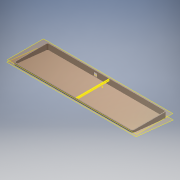
# Autodesk Inventor part: FullEnclosurePrototype
Saved by Autodesk Inventor 2016 (Build 200138000, 138)
## iProperties
Created: 2021-04-05
Part Number: FullEnclosurePrototype
Material: Generic
Document SubType Name: Modeling
Designer: Tom
Density: 1 g/cm^3
Appearance: Default
Author: Tom
Autodesk Inventor part; units mm, degrees
ref_plane "YZ Plane" through (0, 0, 0) normal (1, 0, 0) x (0, 1, 0)
ref_plane "XZ Plane" through (0, 0, 0) normal (0, 1, 0) x (-1, 0, 0)
ref_plane "XY Plane" through (0, 0, 0) normal (0, 0, 1) x (1, 0, 0)
sketch "Sketch1" plane through (0, 0, 0) normal (1, 0, 0) x (0, 1, 0)
  line L0 (-93.1541, 14.0981) -> (20.8459, 14.0981) projected
  line L1 (-93.1541, 14.0981) -> (-93.1541, 12.5981) projected
  line L2 (20.8459, 12.5981) -> (-93.1541, 12.5981) projected
  line L3 (20.8459, 14.0981) -> (20.8459, 12.5981) projected
  line L4 (-93.1541, 7.4943) -> (-93.1541, 9.0943) projected
  line L5 (-93.1541, 7.4943) -> (20.8459, 7.4943) projected
  line L6 (20.8459, 7.4943) -> (20.8459, 9.0943) projected
  line L7 (-93.1541, 9.0943) -> (20.8459, 9.0943) projected
  line L8 (25.5959, 14.0981) -> (20.8459, 14.0981) projected
  line L9 (20.8459, 12.5981) -> (25.5959, 12.5981) projected
  line L10 (25.5959, 14.0981) -> (25.5959, 12.5981) projected
  line L11 (25.5959, 9.0943) -> (20.8459, 9.0943) projected
  line L12 (25.5959, 7.4943) -> (20.8459, 7.4943) projected
  line L13 (25.5959, 7.4943) -> (25.5959, 9.0943) projected
  line L14 (-93.1541, 9.0943) -> (-97.9041, 9.0943) projected
  line L15 (-93.1541, 7.4943) -> (-97.9041, 7.4943) projected
  line L16 (-97.9041, 7.4943) -> (-97.9041, 9.0943) projected
  line L17 (-93.1541, 14.0981) -> (-97.9041, 14.0981) projected
  line L18 (-97.9041, 12.5981) -> (-93.1541, 12.5981) projected
  line L19 (-97.9041, 14.0981) -> (-97.9041, 12.5981) projected
  line L20 (-93.4041, 11.6343) -> (-93.3041, 11.6343) projected
  point P0 (0, 0)
ref_plane "Work Plane1" through (-45.4451, 14.3376, -5.5632) normal (0, 0.1062088, 0.9943439) x (-1, 0, 0)
ref_plane "Work Plane2" through (-9.3413, -36.1541, 14.0981) normal (0, 0, 1) x (1, 0, 0)
sketch "Sketch3" plane through (-9.3413, -36.1541, 14.0981) normal (0, 0, 1) x (1, 0, 0)
  line L0 (-211.6644, 41.535) -> (-205.2313, 59.21) projected
  line L1 (-205.2313, 59.21) -> (-202.7313, 59.21) projected
  line L2 (-202.7313, 59.21) -> (-209.1644, 41.535) projected
  line L3 (-209.1644, 41.535) -> (-211.6644, 41.535) projected
  line L4 (-201.6644, 41.535) -> (-195.2313, 59.21) projected
  line L5 (-195.2313, 59.21) -> (-192.7313, 59.21) projected
  line L6 (-192.7313, 59.21) -> (-199.1644, 41.535) projected
  line L7 (-199.1644, 41.535) -> (-201.6644, 41.535) projected
  line L8 (-191.6644, 41.535) -> (-185.2313, 59.21) projected
  line L9 (-185.2313, 59.21) -> (-182.7313, 59.21) projected
  line L10 (-182.7313, 59.21) -> (-189.1644, 41.535) projected
  line L11 (-189.1644, 41.535) -> (-191.6644, 41.535) projected
  line L12 (-181.6644, 41.535) -> (-175.2313, 59.21) projected
  line L13 (-175.2313, 59.21) -> (-172.7313, 59.21) projected
  line L14 (-172.7313, 59.21) -> (-179.1644, 41.535) projected
  line L15 (-179.1644, 41.535) -> (-181.6644, 41.535) projected
  line L16 (-171.6644, 41.535) -> (-165.2313, 59.21) projected
  line L17 (-165.2313, 59.21) -> (-162.7313, 59.21) projected
  line L18 (-162.7313, 59.21) -> (-169.1644, 41.535) projected
  line L19 (-169.1644, 41.535) -> (-171.6644, 41.535) projected
  line L20 (-161.6644, 41.535) -> (-155.2313, 59.21) projected
  line L21 (-155.2313, 59.21) -> (-152.7313, 59.21) projected
  line L22 (-152.7313, 59.21) -> (-159.1644, 41.535) projected
  line L23 (-159.1644, 41.535) -> (-161.6644, 41.535) projected
  line L24 (-151.6644, 41.535) -> (-145.2313, 59.21) projected
  line L25 (-145.2313, 59.21) -> (-142.7313, 59.21) projected
  line L26 (-142.7313, 59.21) -> (-149.1644, 41.535) projected
  line L27 (-149.1644, 41.535) -> (-151.6644, 41.535) projected
  line L28 (-141.6644, 41.535) -> (-135.2313, 59.21) projected
  line L29 (-135.2313, 59.21) -> (-132.7313, 59.21) projected
  line L30 (-132.7313, 59.21) -> (-139.1644, 41.535) projected
  line L31 (-139.1644, 41.535) -> (-141.6644, 41.535) projected
  line L32 (-134.1647, 41.535) -> (-136.6647, 41.535) projected
  line L33 (-136.6647, 41.535) -> (-131.39, 56.027) projected
  line L34 (-131.39, 56.027) -> (-131.39, 49.1583) projected
  line L35 (-131.39, 49.1583) -> (-134.1647, 41.535) projected
  line L36 (-141.27, 35.75) -> (-143.77, 35.75) projected
  line L37 (-143.77, 35.75) -> (-142.3378, 39.685) projected
  line L38 (-142.3378, 39.685) -> (-139.8378, 39.685) projected
  line L39 (-139.8378, 39.685) -> (-141.27, 35.75) projected
  line L40 (-151.27, 35.75) -> (-153.77, 35.75) projected
  line L41 (-153.77, 35.75) -> (-152.3378, 39.685) projected
  line L42 (-152.3378, 39.685) -> (-149.8378, 39.685) projected
  line L43 (-149.8378, 39.685) -> (-151.27, 35.75) projected
  line L44 (-161.27, 35.75) -> (-163.77, 35.75) projected
  line L45 (-163.77, 35.75) -> (-162.3378, 39.685) projected
  line L46 (-162.3378, 39.685) -> (-159.8378, 39.685) projected
  line L47 (-159.8378, 39.685) -> (-161.27, 35.75) projected
  line L48 (-171.27, 35.75) -> (-173.77, 35.75) projected
  line L49 (-173.77, 35.75) -> (-172.3378, 39.685) projected
  line L50 (-172.3378, 39.685) -> (-169.8378, 39.685) projected
  line L51 (-169.8378, 39.685) -> (-171.27, 35.75) projected
  line L52 (-181.27, 35.75) -> (-183.77, 35.75) projected
  line L53 (-183.77, 35.75) -> (-182.3378, 39.685) projected
  line L54 (-182.3378, 39.685) -> (-179.8378, 39.685) projected
  line L55 (-179.8378, 39.685) -> (-181.27, 35.75) projected
  line L56 (-191.27, 35.75) -> (-193.77, 35.75) projected
  line L57 (-193.77, 35.75) -> (-192.3378, 39.685) projected
  line L58 (-192.3378, 39.685) -> (-189.8378, 39.685) projected
  line L59 (-189.8378, 39.685) -> (-191.27, 35.75) projected
  line L60 (-201.27, 35.75) -> (-203.77, 35.75) projected
  line L61 (-203.77, 35.75) -> (-202.3378, 39.685) projected
  line L62 (-202.3378, 39.685) -> (-199.8378, 39.685) projected
  line L63 (-199.8378, 39.685) -> (-201.27, 35.75) projected
  line L64 (-211.27, 35.75) -> (-213.77, 35.75) projected
  line L65 (-213.77, 35.75) -> (-212.3378, 39.685) projected
  line L66 (-212.3378, 39.685) -> (-209.8378, 39.685) projected
  line L67 (-209.8378, 39.685) -> (-211.27, 35.75) projected
  line L68 (-206.27, 35.75) -> (-208.77, 35.75) projected
  line L69 (-208.77, 35.75) -> (-207.3378, 39.685) projected
  line L70 (-207.3378, 39.685) -> (-204.8378, 39.685) projected
  line L71 (-204.8378, 39.685) -> (-206.27, 35.75) projected
  line L72 (-196.27, 35.75) -> (-198.77, 35.75) projected
  line L73 (-198.77, 35.75) -> (-197.3378, 39.685) projected
  line L74 (-197.3378, 39.685) -> (-194.8378, 39.685) projected
  line L75 (-194.8378, 39.685) -> (-196.27, 35.75) projected
  line L76 (-186.27, 35.75) -> (-188.77, 35.75) projected
  line L77 (-188.77, 35.75) -> (-187.3378, 39.685) projected
  line L78 (-187.3378, 39.685) -> (-184.8378, 39.685) projected
  line L79 (-184.8378, 39.685) -> (-186.27, 35.75) projected
  line L80 (-176.27, 35.75) -> (-178.77, 35.75) projected
  line L81 (-178.77, 35.75) -> (-177.3378, 39.685) projected
  line L82 (-177.3378, 39.685) -> (-174.8378, 39.685) projected
  line L83 (-174.8378, 39.685) -> (-176.27, 35.75) projected
  line L84 (-166.27, 35.75) -> (-168.77, 35.75) projected
  line L85 (-168.77, 35.75) -> (-167.3378, 39.685) projected
  line L86 (-167.3378, 39.685) -> (-164.8378, 39.685) projected
  line L87 (-164.8378, 39.685) -> (-166.27, 35.75) projected
  line L88 (-156.27, 35.75) -> (-158.77, 35.75) projected
  line L89 (-158.77, 35.75) -> (-157.3378, 39.685) projected
  line L90 (-157.3378, 39.685) -> (-154.8378, 39.685) projected
  line L91 (-154.8378, 39.685) -> (-156.27, 35.75) projected
  line L92 (-146.27, 35.75) -> (-148.77, 35.75) projected
  line L93 (-148.77, 35.75) -> (-147.3378, 39.685) projected
  line L94 (-147.3378, 39.685) -> (-144.8378, 39.685) projected
  line L95 (-144.8378, 39.685) -> (-146.27, 35.75) projected
  line L96 (-136.2702, 35.75) -> (-138.7702, 35.75) projected
  line L97 (-138.7702, 35.75) -> (-137.338, 39.685) projected
  line L98 (-137.338, 39.685) -> (-134.838, 39.685) projected
  line L99 (-134.838, 39.685) -> (-136.2702, 35.75) projected
  line L100 (-213.77, 49.4867) -> (-210.231, 59.21) projected
  line L101 (-210.231, 59.21) -> (-207.731, 59.21) projected
  line L102 (-207.731, 59.21) -> (-213.77, 42.618) projected
  line L103 (-213.77, 42.618) -> (-213.77, 49.4867) projected
  line L104 (-146.6644, 41.535) -> (-140.2313, 59.21) projected
  line L105 (-140.2313, 59.21) -> (-137.7313, 59.21) projected
  line L106 (-137.7313, 59.21) -> (-144.1644, 41.535) projected
  line L107 (-144.1644, 41.535) -> (-146.6644, 41.535) projected
  line L108 (-156.6644, 41.535) -> (-150.2313, 59.21) projected
  line L109 (-150.2313, 59.21) -> (-147.7313, 59.21) projected
  line L110 (-147.7313, 59.21) -> (-154.1644, 41.535) projected
  line L111 (-154.1644, 41.535) -> (-156.6644, 41.535) projected
  line L112 (-166.6644, 41.535) -> (-160.2313, 59.21) projected
  line L113 (-160.2313, 59.21) -> (-157.7313, 59.21) projected
  line L114 (-157.7313, 59.21) -> (-164.1644, 41.535) projected
  line L115 (-164.1644, 41.535) -> (-166.6644, 41.535) projected
  line L116 (-176.6644, 41.535) -> (-170.2313, 59.21) projected
  line L117 (-170.2313, 59.21) -> (-167.7313, 59.21) projected
  line L118 (-167.7313, 59.21) -> (-174.1644, 41.535) projected
  line L119 (-174.1644, 41.535) -> (-176.6644, 41.535) projected
  line L120 (-186.6644, 41.535) -> (-180.2313, 59.21) projected
  line L121 (-180.2313, 59.21) -> (-177.7313, 59.21) projected
  line L122 (-177.7313, 59.21) -> (-184.1644, 41.535) projected
  line L123 (-184.1644, 41.535) -> (-186.6644, 41.535) projected
  line L124 (-196.6644, 41.535) -> (-190.2313, 59.21) projected
  line L125 (-190.2313, 59.21) -> (-187.7313, 59.21) projected
  line L126 (-187.7313, 59.21) -> (-194.1644, 41.535) projected
  line L127 (-194.1644, 41.535) -> (-196.6644, 41.535) projected
  line L128 (-206.6644, 41.535) -> (-200.2313, 59.21) projected
  line L129 (-200.2313, 59.21) -> (-197.7313, 59.21) projected
  line L130 (-197.7313, 59.21) -> (-204.1644, 41.535) projected
  line L131 (-204.1644, 41.535) -> (-206.6644, 41.535) projected
  line L132 (-78.7722, 35.75) -> (-133.77, 35.75) projected
  line L133 (-133.77, 35.75) -> (-132.3378, 39.685) projected
  line L134 (-132.3378, 39.685) -> (-77.34, 39.685) projected
  line L135 (-77.34, 39.685) -> (-78.7722, 35.75) projected
  line L136 (-77.34, 41.535) -> (-129.54, 41.535) projected
  line L137 (-129.54, 41.535) -> (-129.54, 59.315) projected
  line L138 (-129.54, 59.315) -> (-77.34, 59.315) projected
  line L139 (-77.34, 59.315) -> (-77.34, 41.535) projected
  line L140 (159, -26.25) -> (159, -40.25) projected
  line L141 (159, -40.25) -> (145, -40.25) projected
  line L142 (145, -40.25) -> (145, -26.25) projected
  line L143 (145, -26.25) -> (159, -26.25) projected
  line L144 (140, -26.25) -> (140, -40.25) projected
  line L145 (140, -40.25) -> (126, -40.25) projected
  line L146 (126, -40.25) -> (126, -26.25) projected
  line L147 (126, -26.25) -> (140, -26.25) projected
  line L148 (121, -26.25) -> (121, -40.25) projected
  line L149 (121, -40.25) -> (107, -40.25) projected
  line L150 (107, -40.25) -> (107, -26.25) projected
  line L151 (107, -26.25) -> (121, -26.25) projected
  line L152 (102, -26.25) -> (102, -40.25) projected
  line L153 (102, -40.25) -> (88, -40.25) projected
  line L154 (88, -40.25) -> (88, -26.25) projected
  line L155 (88, -26.25) -> (102, -26.25) projected
  line L156 (83, -26.25) -> (83, -40.25) projected
  line L157 (83, -40.25) -> (69, -40.25) projected
  line L158 (69, -40.25) -> (69, -26.25) projected
  line L159 (69, -26.25) -> (83, -26.25) projected
  line L160 (64, -26.25) -> (64, -40.25) projected
  line L161 (64, -40.25) -> (50, -40.25) projected
  line L162 (50, -40.25) -> (50, -26.25) projected
  line L163 (50, -26.25) -> (64, -26.25) projected
  line L164 (45, -26.25) -> (45, -40.25) projected
  line L165 (45, -40.25) -> (31, -40.25) projected
  line L166 (31, -40.25) -> (31, -26.25) projected
  line L167 (31, -26.25) -> (45, -26.25) projected
  line L168 (26, -26.25) -> (26, -40.25) projected
  line L169 (26, -40.25) -> (12, -40.25) projected
  line L170 (12, -40.25) -> (12, -26.25) projected
  line L171 (12, -26.25) -> (26, -26.25) projected
  line L172 (7, -26.25) -> (7, -40.25) projected
  line L173 (7, -40.25) -> (-7, -40.25) projected
  line L174 (-7, -40.25) -> (-7, -26.25) projected
  line L175 (-7, -26.25) -> (7, -26.25) projected
  line L176 (154.5, -7.25) -> (168.5, -7.25) projected
  line L177 (168.5, -7.25) -> (168.5, -21.25) projected
  line L178 (168.5, -21.25) -> (154.5, -21.25) projected
  line L179 (154.5, -21.25) -> (154.5, -7.25) projected
  line L180 (135.5, -7.25) -> (149.5, -7.25) projected
  line L181 (149.5, -7.25) -> (149.5, -21.25) projected
  line L182 (149.5, -21.25) -> (135.5, -21.25) projected
  line L183 (135.5, -21.25) -> (135.5, -7.25) projected
  line L184 (116.5, -7.25) -> (130.5, -7.25) projected
  line L185 (130.5, -7.25) -> (130.5, -21.25) projected
  line L186 (130.5, -21.25) -> (116.5, -21.25) projected
  line L187 (116.5, -21.25) -> (116.5, -7.25) projected
  line L188 (97.5, -7.25) -> (111.5, -7.25) projected
  line L189 (111.5, -7.25) -> (111.5, -21.25) projected
  line L190 (111.5, -21.25) -> (97.5, -21.25) projected
  line L191 (97.5, -21.25) -> (97.5, -7.25) projected
  line L192 (78.5, -7.25) -> (92.5, -7.25) projected
  line L193 (92.5, -7.25) -> (92.5, -21.25) projected
  line L194 (92.5, -21.25) -> (78.5, -21.25) projected
  line L195 (78.5, -21.25) -> (78.5, -7.25) projected
  line L196 (59.5, -7.25) -> (73.5, -7.25) projected
  line L197 (73.5, -7.25) -> (73.5, -21.25) projected
  line L198 (73.5, -21.25) -> (59.5, -21.25) projected
  line L199 (59.5, -21.25) -> (59.5, -7.25) projected
  line L200 (40.5, -7.25) -> (54.5, -7.25) projected
  line L201 (54.5, -7.25) -> (54.5, -21.25) projected
  line L202 (54.5, -21.25) -> (40.5, -21.25) projected
  line L203 (40.5, -21.25) -> (40.5, -7.25) projected
  line L204 (21.5, -7.25) -> (35.5, -7.25) projected
  line L205 (35.5, -7.25) -> (35.5, -21.25) projected
  line L206 (35.5, -21.25) -> (21.5, -21.25) projected
  line L207 (21.5, -21.25) -> (21.5, -7.25) projected
  line L208 (2.5, -7.25) -> (16.5, -7.25) projected
  line L209 (16.5, -7.25) -> (16.5, -21.25) projected
  line L210 (16.5, -21.25) -> (2.5, -21.25) projected
  line L211 (2.5, -21.25) -> (2.5, -7.25) projected
  line L212 (-16.5, -7.25) -> (-2.5, -7.25) projected
  line L213 (-2.5, -7.25) -> (-2.5, -21.25) projected
  line L214 (-2.5, -21.25) -> (-16.5, -21.25) projected
  line L215 (-16.5, -21.25) -> (-16.5, -7.25) projected
  line L216 (182.75, 11.75) -> (182.75, -2.25) projected
  line L217 (182.75, -2.25) -> (168.75, -2.25) projected
  line L218 (168.75, -2.25) -> (168.75, 11.75) projected
  line L219 (168.75, 11.75) -> (182.75, 11.75) projected
  line L220 (163.75, 11.75) -> (163.75, -2.25) projected
  line L221 (163.75, -2.25) -> (149.75, -2.25) projected
  line L222 (149.75, -2.25) -> (149.75, 11.75) projected
  line L223 (149.75, 11.75) -> (163.75, 11.75) projected
  line L224 (144.75, 11.75) -> (144.75, -2.25) projected
  line L225 (144.75, -2.25) -> (130.75, -2.25) projected
  line L226 (130.75, -2.25) -> (130.75, 11.75) projected
  line L227 (130.75, 11.75) -> (144.75, 11.75) projected
  line L228 (125.75, 11.75) -> (125.75, -2.25) projected
  line L229 (125.75, -2.25) -> (111.75, -2.25) projected
  line L230 (111.75, -2.25) -> (111.75, 11.75) projected
  line L231 (111.75, 11.75) -> (125.75, 11.75) projected
  line L232 (106.75, 11.75) -> (106.75, -2.25) projected
  line L233 (106.75, -2.25) -> (92.75, -2.25) projected
  line L234 (92.75, -2.25) -> (92.75, 11.75) projected
  line L235 (92.75, 11.75) -> (106.75, 11.75) projected
  line L236 (87.75, 11.75) -> (87.75, -2.25) projected
  line L237 (87.75, -2.25) -> (73.75, -2.25) projected
  line L238 (73.75, -2.25) -> (73.75, 11.75) projected
  line L239 (73.75, 11.75) -> (87.75, 11.75) projected
  line L240 (68.75, 11.75) -> (68.75, -2.25) projected
  line L241 (68.75, -2.25) -> (54.75, -2.25) projected
  line L242 (54.75, -2.25) -> (54.75, 11.75) projected
  line L243 (54.75, 11.75) -> (68.75, 11.75) projected
  line L244 (49.75, 11.75) -> (49.75, -2.25) projected
  line L245 (49.75, -2.25) -> (35.75, -2.25) projected
  line L246 (35.75, -2.25) -> (35.75, 11.75) projected
  line L247 (35.75, 11.75) -> (49.75, 11.75) projected
  line L248 (30.75, 11.75) -> (30.75, -2.25) projected
  line L249 (30.75, -2.25) -> (16.75, -2.25) projected
  line L250 (16.75, -2.25) -> (16.75, 11.75) projected
  line L251 (16.75, 11.75) -> (30.75, 11.75) projected
  line L252 (11.75, 11.75) -> (11.75, -2.25) projected
  line L253 (11.75, -2.25) -> (-2.25, -2.25) projected
  line L254 (-2.25, -2.25) -> (-2.25, 11.75) projected
  line L255 (-2.25, 11.75) -> (11.75, 11.75) projected
  line L256 (-7.25, 11.75) -> (-7.25, -2.25) projected
  line L257 (-7.25, -2.25) -> (-21.25, -2.25) projected
  line L258 (-21.25, -2.25) -> (-21.25, 11.75) projected
  line L259 (-21.25, 11.75) -> (-7.25, 11.75) projected
  line L260 (-12, -26.25) -> (-12, -40.25) projected
  line L261 (-12, -40.25) -> (-26, -40.25) projected
  line L262 (-26, -40.25) -> (-26, -26.25) projected
  line L263 (-26, -26.25) -> (-12, -26.25) projected
  line L264 (-21.5, -7.25) -> (-21.5, -21.25) projected
  line L265 (-21.5, -21.25) -> (-35.5, -21.25) projected
  line L266 (-35.5, -21.25) -> (-35.5, -7.25) projected
  line L267 (-35.5, -7.25) -> (-21.5, -7.25) projected
  line L268 (-26.25, 11.75) -> (-26.25, -2.25) projected
  line L269 (-26.25, -2.25) -> (-40.25, -2.25) projected
  line L270 (-40.25, -2.25) -> (-40.25, 11.75) projected
  line L271 (-40.25, 11.75) -> (-26.25, 11.75) projected
  line L272 (201.75, 30.75) -> (201.75, 16.75) projected
  line L273 (201.75, 16.75) -> (187.75, 16.75) projected
  line L274 (187.75, 16.75) -> (187.75, 30.75) projected
  line L275 (187.75, 30.75) -> (201.75, 30.75) projected
  line L276 (206.5, 11.75) -> (206.5, -2.25) projected
  line L277 (206.5, -2.25) -> (192.5, -2.25) projected
  line L278 (192.5, -2.25) -> (192.5, 11.75) projected
  line L279 (192.5, 11.75) -> (206.5, 11.75) projected
  line L280 (199.375, -7.25) -> (199.375, -21.25) projected
  line L281 (199.375, -21.25) -> (185.375, -21.25) projected
  line L282 (185.375, -21.25) -> (185.375, -7.25) projected
  line L283 (185.375, -7.25) -> (199.375, -7.25) projected
  line L284 (194.625, -26.25) -> (194.625, -40.25) projected
  line L285 (194.625, -40.25) -> (180.625, -40.25) projected
  line L286 (180.625, -40.25) -> (180.625, -26.25) projected
  line L287 (180.625, -26.25) -> (194.625, -26.25) projected
  line L288 (208.875, -45.25) -> (208.875, -59.25) projected
  line L289 (208.875, -59.25) -> (194.875, -59.25) projected
  line L290 (194.875, -59.25) -> (194.875, -45.25) projected
  line L291 (194.875, -45.25) -> (208.875, -45.25) projected
  line L292 (185.125, -45.25) -> (185.125, -59.25) projected
  line L293 (185.125, -59.25) -> (171.125, -59.25) projected
  line L294 (171.125, -59.25) -> (171.125, -45.25) projected
  line L295 (171.125, -45.25) -> (185.125, -45.25) projected
  line L296 (161.375, -45.25) -> (161.375, -59.25) projected
  line L297 (161.375, -59.25) -> (147.375, -59.25) projected
  line L298 (147.375, -59.25) -> (147.375, -45.25) projected
  line L299 (147.375, -45.25) -> (161.375, -45.25) projected
  line L300 (78.25, -45.25) -> (78.25, -59.25) projected
  line L301 (78.25, -59.25) -> (64.25, -59.25) projected
  line L302 (64.25, -59.25) -> (64.25, -45.25) projected
  line L303 (64.25, -45.25) -> (78.25, -45.25) projected
  line L304 (-4.875, -45.25) -> (-4.875, -59.25) projected
  line L305 (-4.875, -59.25) -> (-18.875, -59.25) projected
  line L306 (-18.875, -59.25) -> (-18.875, -45.25) projected
  line L307 (-18.875, -45.25) -> (-4.875, -45.25) projected
  line L308 (-28.625, -45.25) -> (-28.625, -59.25) projected
  line L309 (-28.625, -59.25) -> (-42.625, -59.25) projected
  line L310 (-42.625, -59.25) -> (-42.625, -45.25) projected
  line L311 (-42.625, -45.25) -> (-28.625, -45.25) projected
  line L312 (-52.375, -45.25) -> (-52.375, -59.25) projected
  line L313 (-52.375, -59.25) -> (-66.375, -59.25) projected
  line L314 (-66.375, -59.25) -> (-66.375, -45.25) projected
  line L315 (-66.375, -45.25) -> (-52.375, -45.25) projected
  line L316 (-42.875, -26.25) -> (-42.875, -40.25) projected
  line L317 (-42.875, -40.25) -> (-56.875, -40.25) projected
  line L318 (-56.875, -40.25) -> (-56.875, -26.25) projected
  line L319 (-56.875, -26.25) -> (-42.875, -26.25) projected
  line L320 (-47.625, -7.25) -> (-47.625, -21.25) projected
  line L321 (-47.625, -21.25) -> (-61.625, -21.25) projected
  line L322 (-61.625, -21.25) -> (-61.625, -7.25) projected
  line L323 (-61.625, -7.25) -> (-47.625, -7.25) projected
  line L324 (-50, 11.75) -> (-50, -2.25) projected
  line L325 (-50, -2.25) -> (-64, -2.25) projected
  line L326 (-64, -2.25) -> (-64, 11.75) projected
  line L327 (-64, 11.75) -> (-50, 11.75) projected
  line L328 (173.25, 30.75) -> (173.25, 16.75) projected
  line L329 (173.25, 16.75) -> (159.25, 16.75) projected
  line L330 (159.25, 16.75) -> (159.25, 30.75) projected
  line L331 (159.25, 30.75) -> (173.25, 30.75) projected
  line L332 (154.25, 30.75) -> (154.25, 16.75) projected
  line L333 (154.25, 16.75) -> (140.25, 16.75) projected
  line L334 (140.25, 16.75) -> (140.25, 30.75) projected
  line L335 (140.25, 30.75) -> (154.25, 30.75) projected
  line L336 (135.25, 30.75) -> (135.25, 16.75) projected
  line L337 (135.25, 16.75) -> (121.25, 16.75) projected
  line L338 (121.25, 16.75) -> (121.25, 30.75) projected
  line L339 (121.25, 30.75) -> (135.25, 30.75) projected
  line L340 (116.25, 30.75) -> (116.25, 16.75) projected
  line L341 (116.25, 16.75) -> (102.25, 16.75) projected
  line L342 (102.25, 16.75) -> (102.25, 30.75) projected
  line L343 (102.25, 30.75) -> (116.25, 30.75) projected
  line L344 (97.25, 30.75) -> (97.25, 16.75) projected
  line L345 (97.25, 16.75) -> (83.25, 16.75) projected
  line L346 (83.25, 16.75) -> (83.25, 30.75) projected
  line L347 (83.25, 30.75) -> (97.25, 30.75) projected
  line L348 (78.25, 30.75) -> (78.25, 16.75) projected
  line L349 (78.25, 16.75) -> (64.25, 16.75) projected
  line L350 (64.25, 16.75) -> (64.25, 30.75) projected
  line L351 (64.25, 30.75) -> (78.25, 30.75) projected
  line L352 (59.25, 30.75) -> (59.25, 16.75) projected
  line L353 (59.25, 16.75) -> (45.25, 16.75) projected
  line L354 (45.25, 16.75) -> (45.25, 30.75) projected
  line L355 (45.25, 30.75) -> (59.25, 30.75) projected
  line L356 (40.25, 30.75) -> (40.25, 16.75) projected
  line L357 (40.25, 16.75) -> (26.25, 16.75) projected
  line L358 (26.25, 16.75) -> (26.25, 30.75) projected
  line L359 (26.25, 30.75) -> (40.25, 30.75) projected
  line L360 (21.25, 30.75) -> (21.25, 16.75) projected
  line L361 (21.25, 16.75) -> (7.25, 16.75) projected
  line L362 (7.25, 16.75) -> (7.25, 30.75) projected
  line L363 (7.25, 30.75) -> (21.25, 30.75) projected
  line L364 (2.25, 30.75) -> (2.25, 16.75) projected
  line L365 (2.25, 16.75) -> (-11.75, 16.75) projected
  line L366 (-11.75, 16.75) -> (-11.75, 30.75) projected
  line L367 (-11.75, 30.75) -> (2.25, 30.75) projected
  line L368 (-16.75, 30.75) -> (-16.75, 16.75) projected
  line L369 (-16.75, 16.75) -> (-30.75, 16.75) projected
  line L370 (-30.75, 16.75) -> (-30.75, 30.75) projected
  line L371 (-30.75, 30.75) -> (-16.75, 30.75) projected
  line L372 (-35.75, 30.75) -> (-35.75, 16.75) projected
  line L373 (-35.75, 16.75) -> (-49.75, 16.75) projected
  line L374 (-49.75, 16.75) -> (-49.75, 30.75) projected
  line L375 (-49.75, 30.75) -> (-35.75, 30.75) projected
  line L376 (-54.75, 30.75) -> (-54.75, 16.75) projected
  line L377 (-54.75, 16.75) -> (-68.75, 16.75) projected
  line L378 (-68.75, 16.75) -> (-68.75, 30.75) projected
  line L379 (-68.75, 30.75) -> (-54.75, 30.75) projected
  line L380 (-92.5, -2.25) -> (-92.5, 11.75) projected
  line L381 (-92.5, 11.75) -> (-78.5, 11.75) projected
  line L382 (-78.5, 11.75) -> (-78.5, -2.25) projected
  line L383 (-78.5, -2.25) -> (-92.5, -2.25) projected
  line L384 (-111.5, -2.25) -> (-111.5, 11.75) projected
  line L385 (-111.5, 11.75) -> (-97.5, 11.75) projected
  line L386 (-97.5, 11.75) -> (-97.5, -2.25) projected
  line L387 (-97.5, -2.25) -> (-111.5, -2.25) projected
  line L388 (-130.5, -2.25) -> (-130.5, 11.75) projected
  line L389 (-130.5, 11.75) -> (-116.5, 11.75) projected
  line L390 (-116.5, 11.75) -> (-116.5, -2.25) projected
  line L391 (-116.5, -2.25) -> (-130.5, -2.25) projected
  line L392 (-92.5, 16.75) -> (-92.5, 30.75) projected
  line L393 (-92.5, 30.75) -> (-78.5, 30.75) projected
  line L394 (-78.5, 30.75) -> (-78.5, 16.75) projected
  line L395 (-78.5, 16.75) -> (-92.5, 16.75) projected
  line L396 (-111.5, 16.75) -> (-111.5, 30.75) projected
  line L397 (-111.5, 30.75) -> (-97.5, 30.75) projected
  line L398 (-97.5, 30.75) -> (-97.5, 16.75) projected
  line L399 (-97.5, 16.75) -> (-111.5, 16.75) projected
  line L400 (-116.5, 30.75) -> (-116.5, 16.75) projected
  line L401 (-116.5, 16.75) -> (-130.5, 16.75) projected
  line L402 (-130.5, 16.75) -> (-130.5, 30.75) projected
  line L403 (-130.5, 30.75) -> (-116.5, 30.75) projected
  line L404 (-97.5, -26.25) -> (-97.5, -40.25) projected
  line L405 (-97.5, -40.25) -> (-111.5, -40.25) projected
  line L406 (-111.5, -40.25) -> (-111.5, -26.25) projected
  line L407 (-111.5, -26.25) -> (-97.5, -26.25) projected
  line L408 (-78.5, -45.25) -> (-78.5, -59.25) projected
  line L409 (-78.5, -59.25) -> (-92.5, -59.25) projected
  line L410 (-92.5, -59.25) -> (-92.5, -45.25) projected
  line L411 (-92.5, -45.25) -> (-78.5, -45.25) projected
  line L412 (-97.5, -45.25) -> (-97.5, -59.25) projected
  line L413 (-97.5, -59.25) -> (-111.5, -59.25) projected
  line L414 (-111.5, -59.25) -> (-111.5, -45.25) projected
  line L415 (-111.5, -45.25) -> (-97.5, -45.25) projected
  line L416 (-116.5, -45.25) -> (-116.5, -59.25) projected
  line L417 (-116.5, -59.25) -> (-130.5, -59.25) projected
  line L418 (-130.5, -59.25) -> (-130.5, -45.25) projected
  line L419 (-130.5, -45.25) -> (-116.5, -45.25) projected
  line L420 (-140.25, -35.75) -> (-140.25, -49.75) projected
  line L421 (-140.25, -49.75) -> (-154.25, -49.75) projected
  line L422 (-154.25, -49.75) -> (-154.25, -35.75) projected
  line L423 (-154.25, -35.75) -> (-140.25, -35.75) projected
  line L424 (-140.25, 2.25) -> (-140.25, -11.75) projected
  line L425 (-140.25, -11.75) -> (-154.25, -11.75) projected
  line L426 (-154.25, -11.75) -> (-154.25, 2.25) projected
  line L427 (-154.25, 2.25) -> (-140.25, 2.25) projected
  line L428 (-140.25, 30.75) -> (-140.25, 16.75) projected
  line L429 (-140.25, 16.75) -> (-154.25, 16.75) projected
  line L430 (-154.25, 16.75) -> (-154.25, 30.75) projected
  line L431 (-154.25, 30.75) -> (-140.25, 30.75) projected
  line L432 (-173.25, -45.25) -> (-159.25, -45.25) projected
  line L433 (-159.25, -45.25) -> (-159.25, -59.25) projected
  line L434 (-159.25, -59.25) -> (-173.25, -59.25) projected
  line L435 (-173.25, -59.25) -> (-173.25, -45.25) projected
  line L436 (-192.25, -45.25) -> (-178.25, -45.25) projected
  line L437 (-178.25, -45.25) -> (-178.25, -59.25) projected
  line L438 (-178.25, -59.25) -> (-192.25, -59.25) projected
  line L439 (-192.25, -59.25) -> (-192.25, -45.25) projected
  line L440 (-211.25, -45.25) -> (-197.25, -45.25) projected
  line L441 (-197.25, -45.25) -> (-197.25, -59.25) projected
  line L442 (-197.25, -59.25) -> (-211.25, -59.25) projected
  line L443 (-211.25, -59.25) -> (-211.25, -45.25) projected
  line L444 (-173.25, -26.25) -> (-159.25, -26.25) projected
  line L445 (-159.25, -26.25) -> (-159.25, -40.25) projected
  line L446 (-159.25, -40.25) -> (-173.25, -40.25) projected
  line L447 (-173.25, -40.25) -> (-173.25, -26.25) projected
  line L448 (-192.25, -26.25) -> (-178.25, -26.25) projected
  line L449 (-178.25, -26.25) -> (-178.25, -40.25) projected
  line L450 (-178.25, -40.25) -> (-192.25, -40.25) projected
  line L451 (-192.25, -40.25) -> (-192.25, -26.25) projected
  line L452 (-211.25, -26.25) -> (-197.25, -26.25) projected
  line L453 (-197.25, -26.25) -> (-197.25, -40.25) projected
  line L454 (-197.25, -40.25) -> (-211.25, -40.25) projected
  line L455 (-211.25, -40.25) -> (-211.25, -26.25) projected
  line L456 (-173.25, -7.25) -> (-159.25, -7.25) projected
  line L457 (-159.25, -7.25) -> (-159.25, -21.25) projected
  line L458 (-159.25, -21.25) -> (-173.25, -21.25) projected
  line L459 (-173.25, -21.25) -> (-173.25, -7.25) projected
  line L460 (-192.25, -7.25) -> (-178.25, -7.25) projected
  line L461 (-178.25, -7.25) -> (-178.25, -21.25) projected
  line L462 (-178.25, -21.25) -> (-192.25, -21.25) projected
  line L463 (-192.25, -21.25) -> (-192.25, -7.25) projected
  line L464 (-211.25, -7.25) -> (-197.25, -7.25) projected
  line L465 (-197.25, -7.25) -> (-197.25, -21.25) projected
  line L466 (-197.25, -21.25) -> (-211.25, -21.25) projected
  line L467 (-211.25, -21.25) -> (-211.25, -7.25) projected
  line L468 (-173.25, 11.75) -> (-159.25, 11.75) projected
  line L469 (-159.25, 11.75) -> (-159.25, -2.25) projected
  line L470 (-159.25, -2.25) -> (-173.25, -2.25) projected
  line L471 (-173.25, -2.25) -> (-173.25, 11.75) projected
  line L472 (-192.25, 11.75) -> (-178.25, 11.75) projected
  line L473 (-178.25, 11.75) -> (-178.25, -2.25) projected
  line L474 (-178.25, -2.25) -> (-192.25, -2.25) projected
  line L475 (-192.25, -2.25) -> (-192.25, 11.75) projected
  line L476 (-211.25, 11.75) -> (-197.25, 11.75) projected
  line L477 (-197.25, 11.75) -> (-197.25, -2.25) projected
  line L478 (-197.25, -2.25) -> (-211.25, -2.25) projected
  line L479 (-211.25, -2.25) -> (-211.25, 11.75) projected
  line L480 (-173.25, 30.75) -> (-159.25, 30.75) projected
  line L481 (-159.25, 30.75) -> (-159.25, 16.75) projected
  line L482 (-159.25, 16.75) -> (-173.25, 16.75) projected
  line L483 (-173.25, 16.75) -> (-173.25, 30.75) projected
  line L484 (-192.25, 30.75) -> (-178.25, 30.75) projected
  line L485 (-178.25, 30.75) -> (-178.25, 16.75) projected
  line L486 (-178.25, 16.75) -> (-192.25, 16.75) projected
  line L487 (-192.25, 16.75) -> (-192.25, 30.75) projected
  line L488 (-197.25, 30.75) -> (-197.25, 16.75) projected
  line L489 (-197.25, 16.75) -> (-211.25, 16.75) projected
  line L490 (-211.25, 16.75) -> (-211.25, 30.75) projected
  line L491 (-211.25, 30.75) -> (-197.25, 30.75) projected
  line L492 (211.25, 59.25) -> (211.25, 45.25) projected
  line L493 (211.25, 45.25) -> (197.25, 45.25) projected
  line L494 (197.25, 45.25) -> (197.25, 59.25) projected
  line L495 (197.25, 59.25) -> (211.25, 59.25) projected
  line L496 (192.25, 59.25) -> (192.25, 45.25) projected
  line L497 (192.25, 45.25) -> (178.25, 45.25) projected
  line L498 (178.25, 45.25) -> (178.25, 59.25) projected
  line L499 (178.25, 59.25) -> (192.25, 59.25) projected
  line L500 (173.25, 59.25) -> (173.25, 45.25) projected
  line L501 (173.25, 45.25) -> (159.25, 45.25) projected
  line L502 (159.25, 45.25) -> (159.25, 59.25) projected
  line L503 (159.25, 59.25) -> (173.25, 59.25) projected
  line L504 (154.25, 59.25) -> (154.25, 45.25) projected
  line L505 (154.25, 45.25) -> (140.25, 45.25) projected
  line L506 (140.25, 45.25) -> (140.25, 59.25) projected
  line L507 (140.25, 59.25) -> (154.25, 59.25) projected
  line L508 (125.75, 59.25) -> (125.75, 45.25) projected
  line L509 (125.75, 45.25) -> (111.75, 45.25) projected
  line L510 (111.75, 45.25) -> (111.75, 59.25) projected
  line L511 (111.75, 59.25) -> (125.75, 59.25) projected
  line L512 (106.75, 59.25) -> (106.75, 45.25) projected
  line L513 (106.75, 45.25) -> (92.75, 45.25) projected
  line L514 (92.75, 45.25) -> (92.75, 59.25) projected
  line L515 (92.75, 59.25) -> (106.75, 59.25) projected
  line L516 (87.75, 59.25) -> (87.75, 45.25) projected
  line L517 (87.75, 45.25) -> (73.75, 45.25) projected
  line L518 (73.75, 45.25) -> (73.75, 59.25) projected
  line L519 (73.75, 59.25) -> (87.75, 59.25) projected
  line L520 (68.75, 59.25) -> (68.75, 45.25) projected
  line L521 (68.75, 45.25) -> (54.75, 45.25) projected
  line L522 (54.75, 45.25) -> (54.75, 59.25) projected
  line L523 (54.75, 59.25) -> (68.75, 59.25) projected
  line L524 (40.25, 59.25) -> (40.25, 45.25) projected
  line L525 (40.25, 45.25) -> (26.25, 45.25) projected
  line L526 (26.25, 45.25) -> (26.25, 59.25) projected
  line L527 (26.25, 59.25) -> (40.25, 59.25) projected
  line L528 (21.25, 59.25) -> (21.25, 45.25) projected
  line L529 (21.25, 45.25) -> (7.25, 45.25) projected
  line L530 (7.25, 45.25) -> (7.25, 59.25) projected
  line L531 (7.25, 59.25) -> (21.25, 59.25) projected
  line L532 (2.25, 59.25) -> (2.25, 45.25) projected
  line L533 (2.25, 45.25) -> (-11.75, 45.25) projected
  line L534 (-11.75, 45.25) -> (-11.75, 59.25) projected
  line L535 (-11.75, 59.25) -> (2.25, 59.25) projected
  line L536 (-16.75, 59.25) -> (-16.75, 45.25) projected
  line L537 (-16.75, 45.25) -> (-30.75, 45.25) projected
  line L538 (-30.75, 45.25) -> (-30.75, 59.25) projected
  line L539 (-30.75, 59.25) -> (-16.75, 59.25) projected
  line L540 (-54.75, 59.25) -> (-54.75, 45.25) projected
  line L541 (-54.75, 45.25) -> (-68.75, 45.25) projected
  line L542 (-68.75, 45.25) -> (-68.75, 59.25) projected
  line L543 (-68.75, 59.25) -> (-54.75, 59.25) projected
  line L544 (216.125, 61.75) -> (-216.125, 61.75) projected
  arc A0 (-216.125, 61.75) -> (-220.875, 57) centre (-216.125, 57) ccw projected
  line L545 (-220.875, 57) -> (-220.875, -57) projected
  arc A1 (-220.875, -57) -> (-216.125, -61.75) centre (-216.125, -57) ccw projected
  line L546 (-216.125, -61.75) -> (216.125, -61.75) projected
  arc A2 (216.125, -61.75) -> (220.875, -57) centre (216.125, -57) ccw projected
  line L547 (220.875, -57) -> (220.875, 57) projected
  arc A3 (220.875, 57) -> (216.125, 61.75) centre (216.125, 57) ccw projected
  line L548 (223.875, 57) -> (223.875, -57)
  arc A4 (216.125, -64.75) -> (223.875, -57) centre (216.125, -57) ccw
  line L549 (216.125, -64.75) -> (-216.125, -64.75)
  arc A5 (-223.875, -57) -> (-216.125, -64.75) centre (-216.125, -57) ccw
  line L550 (-223.875, -57) -> (-223.875, 57)
  arc A6 (-216.125, 64.75) -> (-223.875, 57) centre (-216.125, 57) ccw
  line L551 (-216.125, 64.75) -> (216.125, 64.75)
  arc A7 (223.875, 57) -> (216.125, 64.75) centre (216.125, 57) ccw
  circle A8 centre (133, 57) radius 1.35 projected
  circle A9 centre (187.625, 11.875) radius 1.35 projected
  circle A10 centre (166.25, -40.375) radius 1.35 projected
  circle A11 centre (109.25, 13.49) radius 1.35 projected
  circle A12 centre (76, -23.086) radius 1.35 projected
  circle A13 centre (33.25, 13.49) radius 1.35 projected
  circle A14 centre (-175.75, -23.75) radius 1.35 projected
  circle A15 centre (-175.75, 14.25) radius 1.35 projected
  circle A16 centre (-114, 14.25) radius 1.35 projected
  circle A17 centre (47.5, 57) radius 1.35 projected
  circle A18 centre (-9.5, -24.356) radius 1.35 projected
  circle A19 centre (-73.625, 57) radius 1.35 projected
  circle A20 centre (-45.125, 11.875) radius 1.35 projected
  circle A21 centre (-66.5, -19) radius 1.35 projected
  circle A22 centre (-216.125, 0) radius 1.35 projected
  circle A23 centre (-216.125, 57) radius 1.35 projected
  circle A24 centre (-216.125, -57) radius 1.35 projected
  circle A25 centre (-47.5, -57) radius 1.35 projected
  circle A26 centre (-133.753, -57) radius 1.35 projected
  circle A27 centre (23.75, -57) radius 1.35 projected
  circle A28 centre (118.75, -57) radius 1.35 projected
  circle A29 centre (216.125, -57) radius 1.35 projected
  circle A30 centre (216.125, 0) radius 1.35 projected
  circle A31 centre (216.125, 57) radius 1.35 projected
  point P0 (9.3413, 36.1541)
  dimension "d4" = 3
  constraints: 8 end point, 8 point on circle, 4 centre point, 7 other
  measures "d4" distance between parallel lines of L547 L548
extrude "Extrusion3" add sketch "Sketch3" against normal up to surface contours L548 A4 L549 A5 L550 A6 L551 A7 surface through (-45.4451, 14.3376, -5.5632) normal (0, 0.1062088, 0.9943439)
sketch "Sketch7" plane through (-225.4663, 25.5959, -6.7657) normal (0, -1, 0) x (1, 0, 0)
  line L0 (180.5952, 5.7542) -> (180.5952, 1.7766) projected
  arc A0 (180.5952, 5.7542) -> (180.0212, 6.3283) centre (180.0212, 5.7542) ccw projected
  arc A1 (180.0212, 6.3283) -> (180.5952, 6.9023) centre (180.0212, 6.9023) ccw projected
  line L1 (180.5952, 13.8314) -> (180.5952, 6.9023) projected
  line L2 (180.2625, 13.8314) -> (180.5952, 13.8314) projected
  line L3 (180.2625, 13.8314) -> (180.2625, 14.2073) projected
  line L4 (179.5005, 14.2073) -> (180.2625, 14.2073) projected
  line L5 (179.5005, 13.8314) -> (179.5005, 14.2073) projected
  line L6 (167.6895, 13.8314) -> (179.5005, 13.8314) projected
  line L7 (167.6895, 13.8314) -> (167.6895, 14.2073) projected
  line L8 (166.9275, 14.2073) -> (167.6895, 14.2073) projected
  line L9 (166.9275, 13.8314) -> (166.9275, 14.2073) projected
  line L10 (166.5948, 13.8314) -> (166.9275, 13.8314) projected
  line L11 (166.5948, 13.8314) -> (166.5948, 6.9023) projected
  arc A2 (166.5948, 6.9023) -> (167.1688, 6.3283) centre (167.1688, 6.9023) ccw projected
  arc A3 (167.1688, 6.3283) -> (166.5948, 5.7542) centre (167.1688, 5.7542) ccw projected
  line L12 (166.5948, 5.7542) -> (166.5948, 1.7766) projected
  arc A4 (166.5948, 1.7766) -> (167.1688, 1.2025) centre (167.1688, 1.7766) ccw projected
  line L13 (167.1688, 1.2025) -> (180.0212, 1.2025) projected
  arc A5 (180.0212, 1.2025) -> (180.5952, 1.7766) centre (180.0212, 1.7766) ccw projected
  line L14 (166.5948, 6.9023) -> (166.5948, 5.7542)
  line L15 (166.5948, 13.8314) -> (166.5948, 14.2073)
  line L16 (166.9275, 14.2073) -> (166.5948, 14.2073)
  line L17 (167.6895, 14.2073) -> (179.5005, 14.2073)
  line L18 (180.2625, 14.2073) -> (180.5952, 14.2073)
  line L19 (180.5952, 14.2073) -> (180.5952, 13.8314)
  line L20 (180.5952, 6.9023) -> (180.5952, 5.7542)
  line L21 (180.0212, 1.2025) -> (180.5952, 1.2025)
  line L22 (180.5952, 1.7766) -> (180.5952, 1.2025)
  line L23 (166.5948, 1.7766) -> (166.5948, 1.2025)
  line L24 (167.1688, 1.2025) -> (166.5948, 1.2025)
  point P0 (225.4663, 6.7657)
  constraints: 22 end point, 7 point on line, 4 perpendicular, 4 tangent, 3 collinear
extrude "Extrusion4" cut sketch "Sketch7" against normal blind 22
sketch "Sketch8" plane through (-45.4451, 14.3376, -5.5632) normal (0, 0.1062088, 0.9943439) x (-1, 0, 0)
  ellipse E0 centre (180.0212, -6.5454) end of major axis (180.0212, -11.3224) minor radius 4.75 (180.0212, -11.3224) -> (184.7712, -6.5454) ccw projected
  line L0 (184.7712, -6.5454) -> (184.7712, 108.1031) projected
  ellipse E1 centre (180.0212, 108.1031) end of major axis (180.0212, 103.3261) minor radius 4.75 (184.7712, 108.1031) -> (180.0212, 112.8801) ccw projected
  line L1 (180.0212, 112.8801) -> (-252.2288, 112.8801) projected
  ellipse E2 centre (-252.2288, 108.1031) end of major axis (-252.2288, 112.8801) minor radius 4.75 (-252.2288, 112.8801) -> (-256.9788, 108.1031) ccw projected
  line L2 (-256.9788, 108.1031) -> (-256.9788, -6.5454) projected
  ellipse E3 centre (-252.2288, -6.5454) end of major axis (-252.2288, -1.7683) minor radius 4.75 (-256.9788, -6.5454) -> (-252.2288, -11.3224) ccw projected
  line L3 (-252.2288, -11.3224) -> (180.0212, -11.3224) projected
  ellipse E4 centre (-252.2288, -6.5454) end of major axis (-252.2288, -14.3394) minor radius 7.75 (-259.9788, -6.5454) -> (-252.2288, -14.3394) ccw projected
  line L4 (-259.9788, -6.5454) -> (-259.9788, 108.1031) projected
  ellipse E5 centre (-252.2288, 108.1031) end of major axis (-252.2288, 100.309) minor radius 7.75 (-252.2288, 115.8972) -> (-259.9788, 108.1031) ccw projected
  line L5 (-252.2288, 115.8972) -> (180.0212, 115.8972) projected
  ellipse E6 centre (180.0212, 108.1031) end of major axis (180.0212, 115.8972) minor radius 7.75 (187.7712, 108.1031) -> (180.0212, 115.8972) ccw projected
  line L6 (187.7712, 108.1031) -> (187.7712, -6.5454) projected
  ellipse E7 centre (180.0212, -6.5454) end of major axis (180.0212, 1.2487) minor radius 7.75 (180.0212, -14.3394) -> (187.7712, -6.5454) ccw projected
  line L7 (180.0212, -14.3394) -> (-252.2288, -14.3394) projected
  point P0 (-45.4451, 14.8473)
  constraints: 8 other
extrude "Extrusion5" add sketch "Sketch8" against normal blind 6 contours L3 E3 L2 E2 L1 E1 L0 E0 | L4 E5 L5 E6 L6 E7 L7 E4
body "Solid3"
